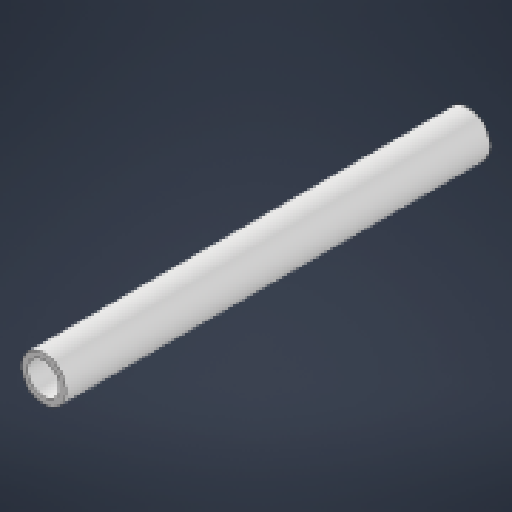
# Autodesk Inventor part: FrameAxlePVC
Saved by Autodesk Inventor 2024.1 (Build 281209000, 209)
## iProperties
Created: 2023-10-16
Part Number: FrameAxlePVC
Material: PVC-Piping
Document SubType Name: Modeling
Designer: Brandon
Density: 1.4 g/cm^3
Appearance: Smooth - White
Author: Brandon
Autodesk Inventor part; units mm, degrees
ref_plane "YZ Plane" through (0, 0, 0) normal (1, 0, 0) x (0, 1, 0)
ref_plane "XZ Plane" through (0, 0, 0) normal (0, 1, 0) x (-1, 0, 0)
ref_plane "XY Plane" through (0, 0, 0) normal (0, 0, 1) x (1, 0, 0)
sketch "Sketch1" plane through (0, 0, 0) normal (0, 0, 1) x (1, 0, 0)
  circle A0 centre (0, 0) radius 10.668
  circle A1 centre (0, 0) radius 7.6454
  dimension "d0" = 21.336
  dimension "d1" = 15.2908
  constraints: 2 centre point, 2 coincident
  measures "d0" diameter of A0
  measures "d1" diameter of A1
extrude "Extrusion1" add sketch "Sketch1" along normal blind 203.2
body "Solid1"
